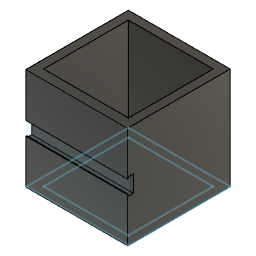
60x10x3 v2 (Autodesk Fusion 360 design; units mm, degrees)
Autodesk Fusion 360 part; units mm, degrees
sketch "Sketch1" plane through (0, 0, 0) normal (0, 0, 1) x (1, 0, 0)
  line L0 (50.6391, 82.0886) -> (110.6391, 82.0886)
  line L1 (110.6391, 82.0886) -> (110.6391, 22.0886)
  line L2 (110.6391, 22.0886) -> (50.6391, 22.0886)
  line L3 (50.6391, 22.0886) -> (50.6391, 82.0886)
  line L4 (55.6391, 77.0886) -> (105.6391, 77.0886)
  line L5 (105.6391, 77.0886) -> (105.6391, 27.0886)
  line L6 (105.6391, 27.0886) -> (55.6391, 27.0886)
  line L7 (55.6391, 27.0886) -> (55.6391, 77.0886)
  dimension "d1" = 60
  dimension "d2" = 60
  dimension "d5" = 50
  dimension "d6" = 50
  constraint horizontal L0
  constraint vertical L1
  constraint horizontal L2
  constraint vertical L3
  constraint horizontal L4
  constraint vertical L5
  constraint horizontal L6
  constraint vertical L7
  measures "d1" distance of L0.start L0.end
  measures "d2" distance of L0.start L2.end
  measures "d5" distance of L4.start L4.end
  measures "d6" distance of L4.start L6.end
extrude "Extrude1" add sketch "Sketch1" along normal blind 10 contours L4 L5 L6 L7
extrude "Extrude2" add sketch "Sketch1" along normal blind 60
sketch "Sketch2" plane through (0, 22.0886, 0) normal (0, -1, 0) x (1, 0, 0)
  line L0 (50.6391, 0) -> (110.6391, 0)
  line L1 (110.6391, 0) -> (110.6391, 60)
  line L2 (110.6391, 60) -> (50.6391, 60)
  line L3 (50.6391, 60) -> (50.6391, 0)
  line L4 (80.6391, 35) -> (75.6391, 35)
  line L5 (75.6391, 35) -> (85.6391, 35)
  line L6 (85.6391, 35) -> (85.6391, 25)
  line L7 (85.6391, 25) -> (75.6391, 25)
  line L8 (75.6391, 25) -> (75.6391, 35)
  dimension "d13" = 10
  dimension "d14" = 10
  constraint horizontal L5
  constraint vertical L6
  constraint horizontal L7
  constraint vertical L8
  measures "d13" distance of L4.end L5.end
  measures "d14" distance of L4.end L7.end
extrude "Extrude3" cut sketch "Sketch2" against normal blind 3.3 contours L4 L5 L6 L7 L8
extrude "Extrude4" add 1 faces at (78.9724, 25.3886, 31.6667) along direction (0, -1, 0) blind 3.3
sketch "Sketch3" plane through (0, 22.0886, 0) normal (0, -1, 0) x (1, 0, 0)
  line L0 (50.6391, 0) -> (110.6391, 0)
  line L1 (110.6391, 0) -> (110.6391, 60)
  line L2 (110.6391, 60) -> (50.6391, 60)
  line L3 (50.6391, 60) -> (50.6391, 0)
extrude "Extrude5" add 1 faces at (70.6391, 22.0886, 40) along direction (0, -1, 0) blind 0.5
sketch "Sketch4" plane through (110.6391, 0, 0) normal (1, 0, 0) x (0, 1, 0)
  line L0 (21.5886, 0) -> (82.0886, 0)
  line L1 (82.0886, 0) -> (82.0886, 60)
  line L2 (82.0886, 60) -> (21.5886, 60)
  line L3 (21.5886, 60) -> (21.5886, 0)
  line L4 (22.0886, 30) -> (22.0886, 35)
  line L5 (22.0886, 35) -> (25.0886, 35)
  line L6 (25.0886, 35) -> (25.0886, 25)
  line L7 (25.0886, 25) -> (22.0886, 25)
  line L8 (22.0886, 25) -> (22.0886, 35)
  line L9 (22.0886, 35) -> (22.0886, 34)
  line L10 (22.0886, 34) -> (21.5886, 34)
  line L11 (21.5886, 34) -> (21.5886, 26)
  line L12 (21.5886, 26) -> (22.0886, 26)
  line L13 (22.0886, 26) -> (22.0886, 34)
  dimension "d22" = 5
  dimension "d23" = 3
  dimension "d24" = 10
  dimension "d25" = 1
  dimension "d26" = 8
  constraint vertical L4
  constraint horizontal L5
  constraint vertical L6
  constraint horizontal L7
  constraint vertical L8
  constraint perpendicular L5 L9
  constraint horizontal L10
  constraint vertical L11
  constraint horizontal L12
  constraint vertical L13
  measures "d22" distance of L4.start L4.end
  measures "d23" distance of L4.end L5.end
  measures "d24" distance of L4.end L7.end
  measures "d25" distance of L4.end L9.end
  measures "d26" distance of L9.end L12.end
extrude "Extrude6" cut sketch "Sketch4" against normal blind 60 contours L3 L4 L8 L10 L11 L12 L13 | L4 L5 L6 L7 L8 L9 L13
